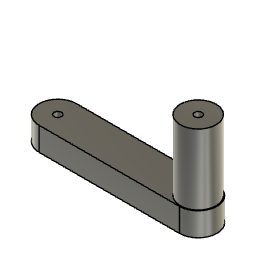
Proximal arm v1 (Autodesk Fusion 360 design; units mm, degrees)
Autodesk Fusion 360 part; units mm, degrees
sketch "Sketch1" plane through (0, 0, 0) normal (0, 0, 1) x (1, 0, 0)
  circle A0 centre (0, 0) radius 20
  line L0 (0, -20) -> (150, -20)
  line L1 (150, -20) -> (150, 20)
  line L2 (150, 20) -> (0, 20)
  line L3 (0, 20) -> (0, -20)
  circle A1 centre (150, 0) radius 20
  dimension "d1" = 40
  dimension "d2" = 150
  constraint coincident A0.centre origin
  constraint horizontal L0
  constraint vertical L1
  constraint horizontal L2
  constraint vertical L3
  constraint coincident A0 L0.start
  constraint midpoint L1 A1.centre
  constraint coincident L1.end A1
  measures "d1" distance of L0.start L2.end
  measures "d2" distance of L0.start L0.end
extrude "Extrude1" add sketch "Sketch1" along normal blind 25
sketch "Sketch2" plane through (0, 0, 0) normal (0, 0, 1) x (1, 0, 0)
  line L0 (13.5959, -7.6257) -> (13.402, 7.9616)
  line L1 (13.402, 7.9616) -> (-0.1939, 15.5873)
  line L2 (-0.1939, 15.5873) -> (-13.5959, 7.6257)
  line L3 (-13.5959, 7.6257) -> (-13.402, -7.9616)
  line L4 (-13.402, -7.9616) -> (0.1939, -15.5873)
  line L5 (0.1939, -15.5873) -> (13.5959, -7.6257)
  circle A0 centre (0, 0) radius 4
  dimension "d5" = 13.5
  dimension "d6" = 8
  constraint coincident A0.centre origin
  measures "d5" distance of A0.centre L5
  measures "d6" diameter of A0
extrude "Extrude2" cut sketch "Sketch2" along normal through all contours A0
sketch "Sketch3" plane through (0, 0, 0) normal (0, 0, 1) x (1, 0, 0)
  circle A0 centre (150, 0) radius 19.082
extrude "Extrude3" add sketch "Sketch3" along normal blind 100
sketch "Sketch4" plane through (0, 0, 0) normal (0, 0, 1) x (1, 0, 0)
  circle A0 centre (150, 0) radius 4
  circle A1 centre (150, 0) radius 4
  dimension "d10" = 8
  dimension "d11" = 8
  constraint concentric A0 A1
  measures "d10" diameter of A0
  measures "d11" diameter of A1
extrude "Extrude4" cut sketch "Sketch4" along normal through all
sketch "Sketch5" plane through (0, 0, 0) normal (0, 0, 1) x (1, 0, 0)
  circle A0 centre (150, 0) radius 10
  circle A1 centre (150, 10) radius 1.5
  point P0 (141.3397, -5)
  point P1 (158.6603, -5)
  dimension "d13" = 3
  dimension "d15" = 360
  constraint coincident A0 A1.centre
  measures "d13" diameter of A1
extrude "Extrude5" cut sketch "Sketch5" 1 faces at (51.2741, 13.7263, 0) against normal blind 3
sketch "Sketch6" plane through (0, 0, 0) normal (0, 0, 1) x (1, 0, 0)
  circle A0 centre (150, 0) radius 10
  circle A1 centre (150, 10) radius 1.5
  point P0 (141.3397, -5)
  point P1 (158.6603, -5)
  dimension "d18" = 3
  dimension "d20" = 360
  constraint coincident A0 A1.centre
  measures "d18" diameter of A1
extrude "Extrude6" cut sketch "Sketch6" along normal blind 3 contours A0 A1 | A0 A1 picked at (150, 9.4917) picked at (149.9812, 10.4913)
sketch "Sketch7" plane through (0, 0, 0) normal (0, 0, 1) x (1, 0, 0)
  circle A0 centre (150, 0) radius 10
  circle A1 centre (150, 10) radius 1.5
  circle A2 centre (158.6603, -5) radius 1.5
  circle A3 centre (141.3397, -5) radius 1.5
  point P0 (141.3397, -5)
  point P1 (158.6603, -5)
  dimension "d23" = 3
  dimension "d25" = 360
  dimension "d26" = 3
  dimension "d27" = 3
  constraint coincident A0 A1.centre
  constraint coincident P1 A2.centre
  constraint coincident P0 A3.centre
  measures "d23" diameter of A1
  measures "d26" diameter of A2
  measures "d27" diameter of A3
extrude "Extrude7" cut sketch "Sketch7" along normal blind 3 contours A0 A1 | A0 A1 | A0 A2 | A0 A2 | A0 A3 | A0 A3
sketch "Sketch8" plane through (0, 0, 0) normal (0, 0, 1) x (1, 0, 0)
  line L0 (-7.7942, 13.5) -> (-15.5885, 0)
  line L1 (-15.5885, 0) -> (-7.7942, -13.5)
  line L2 (-7.7942, -13.5) -> (7.7942, -13.5)
  line L3 (7.7942, -13.5) -> (15.5885, 0)
  line L4 (15.5885, 0) -> (7.7942, 13.5)
  line L5 (7.7942, 13.5) -> (-7.7942, 13.5)
  dimension "d30" = 13.5
  measures "d30" distance of origin L5
extrude "Extrude8" cut sketch "Sketch8" along normal blind 6.35
